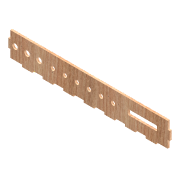
# Autodesk Inventor part: achterzijde elektrobox v2
Saved by Autodesk Inventor 2020.3 (Build 243373000, 373)
## iProperties
Created: 2020-11-26
Part Number: achterzijde elektrobox v2
Material: Wood (Birch)
Document SubType Name: Sheet Metal
Designer: Svend
Density: 0.55 g/cm^3
Sheet Metal Rule: Default_mm
Appearance: Birch - Natural Polished
Author: Svend
Autodesk Inventor part; units mm, degrees
ref_plane "YZ Plane" through (0, 0, 0) normal (1, 0, 0) x (0, 1, 0)
ref_plane "XZ Plane" through (0, 0, 0) normal (0, 1, 0) x (-1, 0, 0)
ref_plane "XY Plane" through (0, 0, 0) normal (0, 0, 1) x (1, 0, 0)
ref_plane "Work Plane1" through (0, 0, 0) normal (0, 0, 1) x (1, 0, 0)
sketch "Sketch1" plane through (0, 0, 0) normal (0, 0, 1) x (1, 0, 0)
  line L0 (-34, 6) -> (-34, 0)
  line L1 (-34, 0) -> (0, 0)
  line L2 (0, 0) -> (0, 6)
  line L3 (0, 6) -> (-34, 6)
  line L4 (0, 6) -> (30, 6)
  line L5 (0, 0) -> (0, 6)
  line L6 (30, 0) -> (0, 0)
  line L7 (30, 0) -> (30, 6)
  line L8 (30, 6) -> (30, 0)
  line L9 (30, 0) -> (60, 0)
  line L10 (60, 0) -> (60, 6)
  line L11 (60, 6) -> (30, 6)
  line L12 (60, 6) -> (90, 6)
  line L13 (60, 0) -> (60, 6)
  line L14 (90, 0) -> (60, 0)
  line L15 (90, 0) -> (90, 6)
  line L16 (90, 6) -> (90, 0)
  line L17 (90, 0) -> (120, 0)
  line L18 (120, 0) -> (120, 6)
  line L19 (120, 6) -> (90, 6)
  line L20 (120, 6) -> (150, 6)
  line L21 (120, 0) -> (120, 6)
  line L22 (150, 0) -> (120, 0)
  line L23 (150, 0) -> (150, 6)
  line L24 (150, 6) -> (150, 0)
  line L25 (150, 0) -> (180, 0)
  line L26 (180, 0) -> (180, 6)
  line L27 (180, 6) -> (150, 6)
  line L28 (180, 6) -> (210, 6)
  line L29 (180, 6) -> (210, 6)
  line L30 (180, 0) -> (180, 6)
  line L31 (210, 0) -> (180, 0)
  line L32 (210, 0) -> (210, 6)
  line L33 (240, 0) -> (240, 6)
  line L34 (240, 6) -> (210, 6)
  line L35 (210, 6) -> (210, 0)
  line L36 (210, 0) -> (240, 0)
  line L37 (240, 6) -> (270, 6)
  line L38 (240, 0) -> (240, 6)
  line L39 (270, 0) -> (240, 0)
  line L40 (270, 0) -> (270, 6)
  line L41 (300, 0) -> (300, 6)
  line L42 (300, 6) -> (270, 6)
  line L43 (270, 6) -> (270, 0)
  line L44 (270, 0) -> (300, 0)
  line L45 (300, 6) -> (330, 6)
  line L46 (300, 0) -> (300, 6)
  line L47 (330, 0) -> (300, 0)
  line L48 (330, 0) -> (330, 6)
  line L49 (360, 0) -> (360, 6)
  line L50 (360, 6) -> (330, 6)
  line L51 (330, 6) -> (330, 0)
  line L52 (330, 0) -> (360, 0)
  line L53 (360, 6) -> (390, 6)
  line L54 (360, 0) -> (360, 6)
  line L55 (390, 0) -> (360, 0)
  line L56 (390, 0) -> (390, 6)
  line L57 (424, 0) -> (424, 6)
  line L58 (424, 6) -> (390, 6)
  line L59 (390, 6) -> (390, 0)
  line L60 (390, 0) -> (424, 0)
  line L61 (-34, 6) -> (424, 6)
  line L62 (424, 6) -> (424, 76)
  line L63 (424, 76) -> (-34, 76)
  line L64 (-34, 76) -> (-34, 6)
  line L65 (401, 57.7) -> (300, 57.7)
  line L66 (-34, 53.5) -> (-40, 53.5)
  line L67 (-40, 53.5) -> (-40, 28.5)
  line L68 (-40, 28.5) -> (-34, 28.5)
  line L69 (-34, 28.5) -> (-34, 53.5)
  line L70 (424, 53.5) -> (430, 53.5)
  line L71 (430, 53.5) -> (430, 28.5)
  line L72 (430, 28.5) -> (424, 28.5)
  line L73 (424, 28.5) -> (424, 53.5)
  point P0 (430, 41)
  point P1 (424, 41)
  point P2 (-40, 41)
  point P3 (-34, 41)
  point P4 (-34, 41)
  dimension "d0" = 70
  dimension "d2" = 6
  dimension "d3" = 6
  dimension "d4" = 25
  measures "d0" distance of L61.end L62.end
  measures "d2" distance of L70.start L70.end
  measures "d3" distance of L66.start L66.end
  measures "d4" distance of L66.end L67.end
extrude "Plate1" add sketch "Sketch1" along normal blind 6 contours L64 L63 L62 L58 L53 L50 L45 L42 L37 L34 L28 L27 L20 L19 L12 L11 L4 L3 | L4 L7 L6 L2 | L68 L67 L66 L64 | L12 L15 L14 L10 | L20 L23 L22 L18 | L70 L71 L72 L62 | L28 L32 L31 L26 | L56 L55 L49 L53 | L37 L40 L39 L33 | L48 L47 L41 L45
sketch "Sketch2" plane through (0, 0, 6) normal (0, 0, 1) x (1, 0, 0)
  line L0 (401, 54.6) -> (401, 8.8) projected
  line L1 (401, 54.6) -> (300, 54.6) projected
  line L2 (300, 8.8) -> (300, 54.6) projected
  line L3 (401, 8.8) -> (300, 8.8) projected
  line L4 (262.8, 9.6) -> (262.8, 15.6) projected
  line L5 (258.8, 15.6) -> (258.8, 9.6) projected
  line L6 (262.8, 15.6) -> (258.8, 15.6) projected
  line L7 (-40, 53.5) -> (-34, 53.5) projected
  line L8 (-40, 28.5) -> (-40, 53.5) projected
  line L9 (-34, 28.5) -> (-40, 28.5) projected
  line L10 (-34, 6) -> (-34, 28.5) projected
  line L11 (0, 6) -> (-34, 6) projected
  line L12 (0, 0) -> (0, 6) projected
  line L13 (30, 0) -> (0, 0) projected
  line L14 (30, 6) -> (30, 0) projected
  line L15 (60, 6) -> (30, 6) projected
  line L16 (60, 0) -> (60, 6) projected
  line L17 (90, 0) -> (60, 0) projected
  line L18 (90, 6) -> (90, 0) projected
  line L19 (120, 6) -> (90, 6) projected
  line L20 (120, 0) -> (120, 6) projected
  line L21 (150, 0) -> (120, 0) projected
  line L22 (150, 6) -> (150, 0) projected
  line L23 (180, 6) -> (150, 6) projected
  line L24 (180, 0) -> (180, 6) projected
  line L25 (210, 0) -> (180, 0) projected
  line L26 (210, 6) -> (210, 0) projected
  line L27 (240, 6) -> (210, 6) projected
  line L28 (240, 0) -> (240, 6) projected
  line L29 (270, 0) -> (240, 0) projected
  line L30 (270, 6) -> (270, 0) projected
  line L31 (300, 6) -> (270, 6) projected
  line L32 (300, 0) -> (300, 6) projected
  line L33 (330, 0) -> (300, 0) projected
  line L34 (330, 6) -> (330, 0) projected
  line L35 (360, 6) -> (330, 6) projected
  line L36 (360, 0) -> (360, 6) projected
  line L37 (390, 0) -> (360, 0) projected
  line L38 (390, 6) -> (390, 0) projected
  line L39 (424, 6) -> (390, 6) projected
  line L40 (424, 28.5) -> (424, 6) projected
  line L41 (430, 28.5) -> (424, 28.5) projected
  line L42 (430, 53.5) -> (430, 28.5) projected
  line L43 (424, 53.5) -> (430, 53.5) projected
  line L44 (424, 76) -> (424, 53.5) projected
  line L45 (-34, 76) -> (424, 76) projected
  line L46 (-34, 53.5) -> (-34, 76) projected
  circle A0 centre (15, 41) radius 8
  line L47 (-40, 28.5) -> (-40, 53.5) projected
  line L48 (308, 48.5) -> (393, 48.5)
  line L49 (393, 48.5) -> (393, 33.5)
  line L50 (393, 33.5) -> (308, 33.5)
  line L51 (308, 33.5) -> (308, 48.5)
  line L52 (308, 48.5) -> (393, 33.5) construction
  line L53 (393, 48.5) -> (308, 33.5) construction
  line L54 (430, 53.5) -> (430, 28.5) projected
  line L55 (90, 0) -> (60, 0) projected
  circle A1 centre (50, 41) radius 8
  circle A2 centre (-20, 41) radius 8
  circle A3 centre (15, 41) radius 8
  circle A4 centre (195, 41) radius 6
  circle A5 centre (230, 41) radius 6
  circle A6 centre (265, 41) radius 6
  circle A7 centre (160, 41) radius 6
  circle A8 centre (195, 41) radius 6
  circle A9 centre (230, 41) radius 6
  circle A10 centre (125, 41) radius 6
  circle A11 centre (160, 41) radius 6
  circle A12 centre (195, 41) radius 6
  circle A13 centre (90, 41) radius 6
  circle A14 centre (125, 41) radius 6
  circle A15 centre (160, 41) radius 6
  point P0 (0, 0)
  point P1 (430, 41)
  point P2 (255, 0)
  point P3 (-40, 41)
  point P4 (15, 0)
  point P5 (350.5, 41)
  point P6 (350.5, 41)
  point P7 (350.5, 41)
  point P8 (350.5, 8.8)
  point P9 (393, 41)
  point P10 (430, 41)
  point P11 (75, 0)
  point P12 (75, 0)
  point P13 (195, 76)
  dimension "d6" = 85
  dimension "d7" = 15
  dimension "d11" = 16
  dimension "d14" = 35
  dimension "d17" = 35
  dimension "d20" = 12
  dimension "d23" = 35
  dimension "d26" = 35
  constraints: 16 centre point, 14 midpoint, 12 end point, 5 horizontal, 3 horizontal alignment, 3 vertical alignment, 2 parallel, 1 coincident, 1 perpendicular, 28 other
  measures "d6" distance of L48.start L48.end
  measures "d7" distance of L48.end L49.end
  measures "d11" diameter of A0
  measures "d14" distance of A0.centre A1.centre
  measures "d17" distance of A0.centre A2.centre
  measures "d20" diameter of A4
  measures "d23" distance of A4.centre A5.centre
  measures "d26" distance of A4.centre A7.centre
extrude "Cut1" cut sketch "Sketch2" against normal blind 6 contours A0 | L48 L49 L50 L51 | A1 | A2 | A4 | A5 | A6 | A7 | A10 | A13
fillet "Corner Round1" radius 3 4 edges at (393, 48.5, 3) (393, 33.5, 3) (308, 48.5, 3) (308, 33.5, 3)
equation "\"d8\" = Thickness"
equation "\"d1\" = Thickness"
equation "\"BendRadius\" = Thickness"
equation "\"BendReliefWidth\" = Thickness"
equation "\"BendReliefDepth\" = 0.5 * Thickness"
equation "\"CornerReliefSize\" = 4 * Thickness"
equation "\"MinimumRemnant\" = 2 * Thickness"
equation "\"TransitionRadius\" = BendRadius"
equation "\"JacobiRadiusSize\" = BendRadius"
equation "\"GapSize\" = Thickness"
equation "\"Thickness\" = 6"
body "Solid1"
